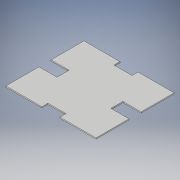
# Autodesk Inventor part: Wood Base
Saved by Autodesk Inventor 2018 (Build 220112000, 112)
## iProperties
Created: 2019-01-03
Part Number: Wood Base
Material: Generic
Document SubType Name: Modeling
Designer: Gabriel
Density: 1 g/cm^3
Appearance: Default
Author: Gabriel
Autodesk Inventor part; units mm, degrees
ref_plane "YZ Plane" through (0, 0, 0) normal (1, 0, 0) x (0, 1, 0)
ref_plane "XZ Plane" through (0, 0, 0) normal (0, 1, 0) x (-1, 0, 0)
ref_plane "XY Plane" through (0, 0, 0) normal (0, 0, 1) x (1, 0, 0)
sketch "Sketch1" plane through (0, 0, 0) normal (0, 1, 0) x (-1, 0, 0)
  line L0 (-212.3768, -878.21) -> (-212.3768, -1157.61)
  line L1 (-212.3768, -1157.61) -> (-364.7768, -1157.61)
  line L2 (-364.7768, -1157.61) -> (-364.7768, -1259.21)
  line L3 (-364.7768, -1259.21) -> (-212.3768, -1259.21)
  line L4 (-212.3768, -1259.21) -> (-212.3768, -1538.61)
  line L5 (-974.3768, -878.21) -> (-974.3768, -1157.61)
  line L6 (-974.3768, -1157.61) -> (-821.9768, -1157.61)
  line L7 (-821.9768, -1157.61) -> (-821.9768, -1259.21)
  line L8 (-821.9768, -1259.21) -> (-974.3768, -1259.21)
  line L9 (-974.3768, -1259.21) -> (-974.3768, -1538.61)
  line L10 (-517.1768, -929.01) -> (-669.5768, -929.01)
  line L11 (-669.5768, -929.01) -> (-669.5768, -878.21)
  line L12 (-517.1768, -929.01) -> (-517.1768, -878.21)
  line L13 (-517.1768, -1538.61) -> (-517.1768, -1487.81)
  line L14 (-517.1768, -1487.81) -> (-669.5768, -1487.81)
  line L15 (-669.5768, -1487.81) -> (-669.5768, -1538.61)
  line L16 (-212.3768, -878.21) -> (-517.1768, -878.21)
  line L17 (-669.5768, -878.21) -> (-974.3768, -878.21)
  line L18 (-212.3768, -1538.61) -> (-517.1768, -1538.61)
  line L19 (-669.5768, -1538.61) -> (-974.3768, -1538.61)
  dimension "d8" = 279.4
  dimension "d9" = 152.4
  dimension "d10" = 101.6
  dimension "d11" = 279.4
  dimension "d12" = 762
  dimension "d13" = 279.4
  dimension "d14" = 152.4
  dimension "d15" = 101.6
  dimension "d16" = 279.4
  dimension "d19" = 152.4
  dimension "d20" = 50.8
  dimension "d22" = 50.8
  dimension "d23" = 152.4
  constraints: 40 end point, 8 perpendicular, 4 point on line, 3 equal length, 2 vertical
  measures "d8" distance of L0.start L0.end
  measures "d9" distance of L0.end L1.end
  measures "d10" distance of L1.end L2.end
  measures "d11" distance of L3.end L4.end
  measures "d12" distance of L0.start L5.start
  measures "d13" distance of L5.start L5.end
  measures "d14" distance of L5.end L6.end
  measures "d15" distance of L6.end L7.end
  measures "d16" distance of L8.end L9.end
  measures "d19" distance of L10.start L10.end
  measures "d20" distance of L10.start L12.end
  measures "d22" distance of L13.start L13.end
  measures "d23" distance of L13.end L14.end
extrude "Wood Base" add sketch "Sketch1" along normal blind 9.525
body "Solid2"
